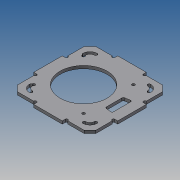
# Autodesk Inventor part: Pieza4
Saved by Autodesk Inventor 2017 (Build 210142000, 142)
## iProperties
Part Number: Pieza4
Material: Genérico
Document SubType Name: Modeling
Designer: Leo
Density: 1 g/cm^3
Appearance: Valor por defecto
Author: Leo
Autodesk Inventor part; units mm, degrees
ref_plane "YZ Plane" through (0, 0, 0) normal (1, 0, 0) x (0, 1, 0)
ref_plane "XZ Plane" through (0, 0, 0) normal (0, 1, 0) x (-1, 0, 0)
ref_plane "XY Plane" through (0, 0, 0) normal (0, 0, 1) x (1, 0, 0)
sketch "Boceto1" plane through (0, 0, 0) normal (0, 0, 1) x (1, 0, 0)
  line L0 (32.5, 7.5) -> (0.5, 7.5) construction
  line L1 (0.5, 7.5) -> (0.5, 31.5) construction
  line L2 (0.5, 31.5) -> (32.5, 31.5) construction
  line L3 (32.5, 31.5) -> (32.5, 7.5) construction
  line L4 (30, -12) -> (30, -31) construction
  line L5 (30, -31) -> (3, -31) construction
  line L6 (3, -31) -> (3, -12) construction
  line L7 (3, -12) -> (30, -12) construction
  line L8 (-59, 20) -> (-59, -20) projected
  line L9 (-59, -20) -> (-55, -20) projected
  arc A0 (-55, -24) -> (-55, -20) centre (-55, -22) ccw projected
  line L10 (-55, -24) -> (-55, -47) projected
  line L11 (-55, -47) -> (-47, -55) projected
  line L12 (-47, -55) -> (-24, -55) projected
  arc A1 (-20, -55) -> (-24, -55) centre (-22, -55) ccw projected
  line L13 (-20, -55) -> (-20, -59) projected
  line L14 (-20, -59) -> (20, -59) projected
  line L15 (20, -59) -> (20, -55) projected
  arc A2 (24, -55) -> (20, -55) centre (22, -55) ccw projected
  line L16 (24, -55) -> (47, -55) projected
  line L17 (47, -55) -> (55, -47) projected
  line L18 (55, -47) -> (55, -24) projected
  arc A3 (55, -20) -> (55, -24) centre (55, -22) ccw projected
  line L19 (55, -20) -> (59, -20) projected
  line L20 (59, -20) -> (59, 20) projected
  line L21 (59, 20) -> (55, 20) projected
  arc A4 (55, 24) -> (55, 20) centre (55, 22) ccw projected
  line L22 (55, 24) -> (55, 47) projected
  line L23 (55, 47) -> (47, 55) projected
  line L24 (47, 55) -> (24, 55) projected
  arc A5 (20, 55) -> (24, 55) centre (22, 55) ccw projected
  line L25 (20, 55) -> (20, 59) projected
  line L26 (20, 59) -> (-20, 59) projected
  line L27 (-20, 59) -> (-20, 55) projected
  arc A6 (-24, 55) -> (-20, 55) centre (-22, 55) ccw projected
  line L28 (-24, 55) -> (-47, 55) projected
  line L29 (-47, 55) -> (-55, 47) projected
  line L30 (-55, 47) -> (-55, 24) projected
  arc A7 (-55, 20) -> (-55, 24) centre (-55, 22) ccw projected
  line L31 (-55, 20) -> (-59, 20) projected
  line L32 (31, 35) -> (-39, 35) construction
  line L33 (-39, 35) -> (-39, -35) construction
  line L34 (-39, -35) -> (31, -35) construction
  line L35 (31, -35) -> (31, 35) construction
  circle A8 centre (31, 35) radius 2
  circle A9 centre (31, -35) radius 2
  circle A10 centre (-39, -35) radius 2
  circle A11 centre (-39, 35) radius 2
  circle A12 centre (-4, 0) radius 32.5
  line L36 (46, 12) -> (46, -12)
  arc A13 (43.6827, -13.9747) -> (46, -12) centre (44, -12) ccw
  line L37 (43.6827, -13.9747) -> (36.6827, -12.85)
  arc A14 (35, -10.8753) -> (36.6827, -12.85) centre (37, -10.8753) ccw
  line L38 (35, -10.8753) -> (35, 10.8753)
  arc A15 (36.6827, 12.85) -> (35, 10.8753) centre (37, 10.8753) ccw
  line L39 (36.6827, 12.85) -> (43.6827, 13.9747)
  arc A16 (46, 12) -> (43.6827, 13.9747) centre (44, 12) ccw
  arc A17 (-37.5, -47.6) -> (-37.5, -43.4) centre (-37.5, -45.5) ccw projected
  arc A18 (-47.6, -37.5) -> (-37.5, -47.6) centre (-37.5, -37.5) ccw projected
  arc A19 (-43.4, -37.5) -> (-47.6, -37.5) centre (-45.5, -37.5) ccw projected
  arc A20 (-43.4, -37.5) -> (-37.5, -43.4) centre (-37.5, -37.5) ccw projected
  arc A21 (-47.6, 37.5) -> (-43.4, 37.5) centre (-45.5, 37.5) ccw projected
  arc A22 (-37.5, 47.6) -> (-47.6, 37.5) centre (-37.5, 37.5) ccw projected
  arc A23 (-37.5, 43.4) -> (-37.5, 47.6) centre (-37.5, 45.5) ccw projected
  arc A24 (-37.5, 43.4) -> (-43.4, 37.5) centre (-37.5, 37.5) ccw projected
  arc A25 (37.5, 47.6) -> (37.5, 43.4) centre (37.5, 45.5) ccw projected
  arc A26 (47.6, 37.5) -> (37.5, 47.6) centre (37.5, 37.5) ccw projected
  arc A27 (43.4, 37.5) -> (47.6, 37.5) centre (45.5, 37.5) ccw projected
  arc A28 (43.4, 37.5) -> (37.5, 43.4) centre (37.5, 37.5) ccw projected
  arc A29 (37.5, -43.4) -> (37.5, -47.6) centre (37.5, -45.5) ccw projected
  arc A30 (37.5, -43.4) -> (43.4, -37.5) centre (37.5, -37.5) ccw projected
  arc A31 (47.6, -37.5) -> (43.4, -37.5) centre (45.5, -37.5) ccw projected
  arc A32 (37.5, -47.6) -> (47.6, -37.5) centre (37.5, -37.5) ccw projected
  point P0 (31, 0)
  point P1 (59, 0)
  point P2 (-4, 35)
  point P3 (35, 0)
  point P4 (46, 0)
  dimension "d0" = 70
  dimension "d1" = 4
  dimension "d2" = 65
  dimension "d3" = 2
  dimension "d4" = 11
  dimension "d5" = 28
  dimension "d6" = 25.7
  dimension "d7" = 16
  dimension "d8" = 4
  constraints: 16 end point, 9 centre point, 8 point on circle, 8 tangent, 6 equal radius, 5 midpoint, 4 coincident, 4 horizontal alignment, 3 parallel, 2 perpendicular, 1 horizontal, 1 vertical, 1 vertical alignment
  measures "d0" distance of L32.start L32.end
  measures "d1" diameter of A8
  measures "d2" diameter of A12
  measures "d3" radius of A15
  measures "d4" distance between parallel lines of L36 L38
  measures "d6" distance of L39.start L37.end
  measures "d7" distance between parallel lines of L33 L30
  measures "d8" distance between parallel lines of L38 L35
extrude "Extrusión1" add sketch "Boceto1" along normal blind 4
